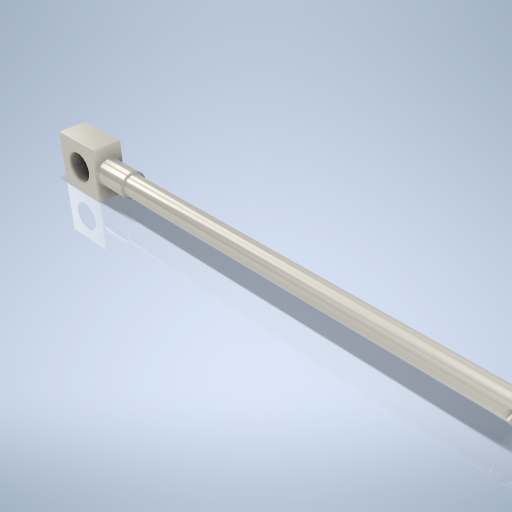
# Autodesk Inventor part: BMS_24
Saved by Autodesk Inventor 2024.2 (Build 282272000, 272)
## iProperties
Created: 2024-05-14
Part Number: BMS_24
Material: Titan
Document SubType Name: Modeling
Designer: Fabri
Density: 4.51 g/cm^3
Appearance: Titan
Author: Fabri
Autodesk Inventor part; units mm, degrees
ref_plane "YZ Plane" through (0, 0, 0) normal (1, 0, 0) x (0, 1, 0)
ref_plane "XY Plane" through (0, 0, 0) normal (0, 0, 1) x (1, 0, 0)
sketch "Skizze1" plane through (0, 0, 0) normal (0, 1, 0) x (-1, 0, 0)
  line L0 (-5, 5) -> (5, 5)
  line L1 (5, 5) -> (5, -5)
  line L2 (5, -5) -> (-5, -5)
  line L3 (-5, -5) -> (-5, 5)
  line L4 (-5, 5) -> (5, -5) construction
  line L5 (5, 5) -> (-5, -5) construction
  point P0 (0, 0)
  dimension "d0" = 10
  dimension "d1" = 10
  constraints: 12 end point, 2 midpoint, 2 parallel, 1 horizontal, 1 perpendicular
  measures "d0" distance of L1.end L2.end
  measures "d1" distance of L0.end L1.end
extrude "Extrusion1" add sketch "Skizze1" along normal mid plane 5.5
sketch "Skizze2" plane through (5, -2.75, -5) normal (1, 0, 0) x (0, 0, -1)
  circle A0 centre (-5, 2.75) radius 2.5
  dimension "d4" = 5
  constraints: 1 centre point, 1 coincident
  measures "d4" diameter of A0
extrude "Extrusion2" add sketch "Skizze2" along normal blind 6.5
sketch "Skizze3" plane through (11.5, 0, 0) normal (1, 0, 0) x (0, 0, -1)
  circle A0 centre (0, 0) radius 2.5 projected
  circle A1 centre (0, 0) radius 2
  dimension "d7" = 4
  constraints: 1 centre point, 1 coincident
  measures "d7" diameter of A1
extrude "Extrusion3" add sketch "Skizze3" along normal blind 74 contours A1
sketch "Skizze4" plane through (0, 2.75, 0) normal (0, 1, 0) x (1, 0, 0)
  point P0 (0, 0)
  point P1 (0, 0)
  constraints: 1 coincident
hole "Bohrung1" at (0, 2.75, 0) direction (0, -1, 0) diameter 5.5 depth 5.5
ref_plane "Arbeitsebene1" through (0, 2, 0) normal (0, 1, 0) x (-1, 0, 0)
sketch "Skizze5" plane through (0, 2, 0) normal (0, 1, 0) x (-1, 0, 0)
  line L0 (-85.5, 2) -> (-85.5, -2) projected
  point P0 (0, 0)
  point P1 (-83, 0)
  dimension "d18" = 2.5
  constraints: 1 horizontal alignment
  measures "d18" distance from line of point (-83, 0) L0
hole "Bohrung2" at (83, 2, 0) direction (0, -1, 0) diameter 2 end through all
chamfer "Fasen1" distance 1 angle 45 1 edges at (85.5, 0, 2)
